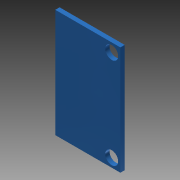
# Autodesk Inventor part: Compass
Saved by Autodesk Inventor 2015 (Build 190159000, 159)
## iProperties
Created: 2016-02-20
Part Number: Compass
Material: Generic
Document SubType Name: Modeling
Designer: 23902
Density: 1 g/cm^3
Appearance: Default
Author: 23902
Autodesk Inventor part; units mm, degrees
ref_plane "YZ Plane" through (0, 0, 0) normal (1, 0, 0) x (0, 1, 0)
ref_plane "XZ Plane" through (0, 0, 0) normal (0, 1, 0) x (-1, 0, 0)
ref_plane "XY Plane" through (0, 0, 0) normal (0, 0, 1) x (1, 0, 0)
sketch "Sketch1" plane through (0, 0, 0) normal (0, 1, 0) x (-1, 0, 0)
  line L0 (-7.5, 12.5) -> (7.5, 12.5)
  line L1 (7.5, 12.5) -> (7.5, -12.5)
  line L2 (7.5, -12.5) -> (-7.5, -12.5)
  line L3 (-7.5, -12.5) -> (-7.5, 12.5)
  line L4 (-7.5, 12.5) -> (7.5, -12.5) construction
  line L5 (7.5, 12.5) -> (4.96, 12.5)
  line L6 (-7.5, 12.5) -> (-5.5, 12.5)
  circle A0 centre (-5.5, 10.5) radius 1.5
  line L7 (-7.5, -12.5) -> (-7.5, -10.5)
  circle A1 centre (-5.5, -10.5) radius 1.5
  point P0 (0, 0)
  dimension "d0" = 15
  dimension "d1" = 25
  dimension "d9" = 2
  dimension "d11" = 3
  dimension "d12" = 2
  dimension "d14" = 3
  constraints: 16 end point, 3 point on line, 2 centre point, 2 parallel, 1 horizontal, 1 midpoint, 1 perpendicular
  measures "d0" distance of L0.start L0.end
  measures "d1" distance of L0.end L1.end
  measures "d9" distance of L0.start L6.end
  measures "d11" diameter of A0
  measures "d12" distance of L2.end L7.end
  measures "d14" diameter of A1
extrude "Extrusion1" add sketch "Sketch1" along normal blind 1
body "Solid1"
